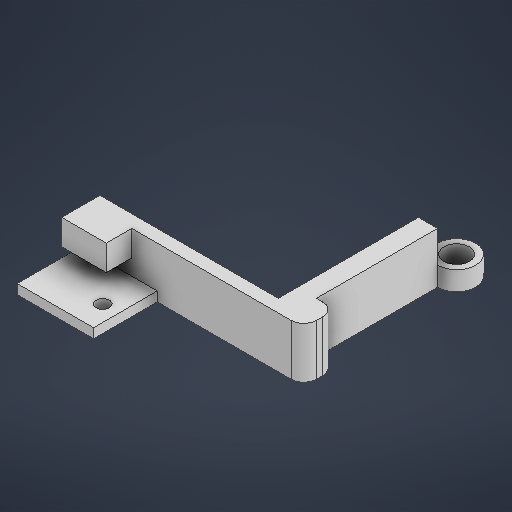
# Autodesk Inventor part: lewascianakoło
Saved by Autodesk Inventor 2026.2 (Build 302298010, 298A)
## iProperties
Created: 2026-04-27
Part Number: lewascianakoło
Material: Ogólny
Document SubType Name: Modeling
Designer: karol
Density: 1 g/cm^3
Appearance: Domyślna
Author: karol
Autodesk Inventor part; units mm, degrees
ref_plane "YZ Plane" through (0, 0, 0) normal (1, 0, 0) x (0, 1, 0)
ref_plane "XZ Plane" through (0, 0, 0) normal (0, 1, 0) x (-1, 0, 0)
ref_plane "XY Plane" through (0, 0, 0) normal (0, 0, 1) x (1, 0, 0)
sketch "Szkic1" plane through (0, 0, 0) normal (0, 1, 0) x (-1, 0, 0)
  line L0 (0, 0) -> (3, 0)
  line L1 (3, 0) -> (3, -25)
  line L2 (3, -25) -> (0, -25)
  line L3 (0, -25) -> (0, 0)
  line L4 (3, 0) -> (31, 0)
  line L5 (31, 0) -> (31, -3)
  line L6 (31, -3) -> (3, -3)
  line L7 (3, -3) -> (3, 0)
  point P0 (3, -3)
  dimension "d0" = 3
  dimension "d1" = 25
  dimension "d2" = 28
  dimension "d3" = 3
  constraints: 16 end point, 4 parallel, 2 horizontal, 2 perpendicular
  measures "d0" distance of L1.end L2.end
  measures "d1" distance of L0.end L1.end
  measures "d2" distance of L5.end L6.end
  measures "d3" distance of L4.end L5.end
extrude "Wyciągnięcie proste1" add sketch "Szkic1" along normal blind 8
sketch "Szkic7" plane through (0, 8, 0) normal (0, 1, 0) x (1, 0, 0)
  line L0 (-31, 0) -> (0, 0) projected
  line L1 (0, 0) -> (-3, 0)
  line L2 (-3, 0) -> (-3, 3)
  line L3 (-3, 3) -> (0, 3)
  line L4 (0, 3) -> (0, 0)
  line L5 (-3, 0) -> (3, 0)
  line L6 (3, 0) -> (3, 6)
  line L7 (3, 6) -> (-3, 6)
  line L8 (-3, 6) -> (-3, 0)
  circle A0 centre (0, 3) radius 1.5
  point P0 (-1.5, 3)
  point P1 (0, 1.5)
  dimension "d21" = 6
  dimension "d22" = 6
  dimension "d23" = 3
  constraints: 16 end point, 4 parallel, 2 horizontal, 2 perpendicular, 1 centre point, 1 coincident
  measures "d21" distance of L7.end L6.end
  measures "d22" distance of L6.end L5.end
  measures "d23" diameter of A0
extrude "Wyciągnięcie proste7" add sketch "Szkic7" against normal blind 8 contours L4 A0 L3 L8 L7 L6 L5
extrude "Wyciągnięcie proste8" cut sketch "Szkic7" against normal blind 8 contours A0 L3 L4 | L4 L3 A0
sketch "Szkic8" plane through (0, 8, 0) normal (0, 1, 0) x (1, 0, 0)
  circle A0 centre (0, 3) radius 1.5 projected
  circle A1 centre (0, 3) radius 2
  point P0 (0, 0)
  constraints: 1 centre point, 1 coincident
extrude "Wyciągnięcie proste9" add sketch "Szkic8" against normal blind 3 contours A0
sketch "Szkic9" plane through (0, 8, 0) normal (0, 1, 0) x (1, 0, 0)
  line L0 (-31, 3) -> (-31, 0) projected
  line L1 (3, 0) -> (3, 6) projected
  line L2 (-31, 0) -> (3, 0)
  line L3 (3, 0) -> (3, 1)
  line L4 (3, 1) -> (-31, 1)
  line L5 (-31, 1) -> (-31, 0)
  point P0 (0, 0)
  dimension "d30" = 1
  constraints: 8 end point, 2 parallel, 1 horizontal, 1 perpendicular, 1 point on line
  measures "d30" distance of L3.end L2.end
extrude "Wyciągnięcie proste10" cut sketch "Szkic9" against normal blind 8
sketch "Szkic10" plane through (0, 8, 0) normal (0, 1, 0) x (1, 0, 0)
  line L0 (0, 25) -> (-3, 25) projected
  line L1 (-3, 25) -> (3, 25)
  line L2 (3, 25) -> (3, 31)
  line L3 (3, 31) -> (-3, 31)
  line L4 (-3, 31) -> (-3, 25)
  point P0 (0, 0)
  dimension "d33" = 6
  dimension "d34" = 6
  constraints: 8 end point, 2 parallel, 1 horizontal, 1 perpendicular
  measures "d33" distance of L3.end L2.end
  measures "d34" distance of L2.end L1.end
extrude "Wyciągnięcie proste11" add sketch "Szkic10" against normal blind 8
sketch "Szkic11" plane through (0, 8, 0) normal (0, 1, 0) x (1, 0, 0)
  line L0 (3, 31) -> (3, 25) projected
  line L1 (3, 31) -> (-3, 31)
  line L2 (-3, 31) -> (-3, 25)
  line L3 (-3, 25) -> (3, 25)
  line L4 (3, 25) -> (3, 31)
  point P0 (0, 0)
  dimension "d37" = 6
  dimension "d38" = 6
  constraints: 8 end point, 2 parallel, 1 horizontal, 1 perpendicular
  measures "d37" distance of L3.end L2.end
  measures "d38" distance of L2.end L1.end
extrude "Wyciągnięcie proste12" cut sketch "Szkic11" against normal blind 5
sketch "Szkic12" plane through (0, 3, 0) normal (0, 1, 0) x (1, 0, 0)
  circle A0 centre (0, 28) radius 2
  line L0 (-3, 25) -> (-3, 31) projected
  line L1 (-3, 31) -> (3, 31) projected
  point P0 (0, 0)
  point P1 (-3, 28)
  point P2 (0, 31)
  dimension "d41" = 4
  dimension "d42" = 3
  dimension "d43" = 3
  constraints: 2 midpoint, 1 centre point
  measures "d41" diameter of A0
  measures "d42" distance of point (-3, 28) A0.centre
  measures "d43" distance of A0.centre point (0, 31)
extrude "Wyciągnięcie proste13" cut sketch "Szkic12" against normal blind 3
sketch "Szkic13" plane through (-31, 8, -1) normal (0, 0, 1) x (1, 0, 0)
  line L0 (0, 0) -> (7, 0)
  line L1 (7, 0) -> (7, -4)
  line L2 (7, -4) -> (0, -4)
  line L3 (0, -4) -> (0, 0)
  point P0 (31, -8)
  dimension "d46" = 7
  dimension "d47" = 4
  constraints: 8 end point, 2 parallel, 1 horizontal, 1 perpendicular
  measures "d46" distance of L1.end L2.end
  measures "d47" distance of L0.end L1.end
extrude "Wyciągnięcie proste14" add sketch "Szkic13" along normal blind 4
sketch "Szkic14" plane through (-31, 0, -3) normal (-1, 0, 0) x (0, 0, 1)
  circle A0 centre (4, 6) radius 1.5
  line L0 (2, 4) -> (6, 4) projected
  line L1 (6, 8) -> (6, 4) projected
  point P0 (3, 0)
  dimension "d50" = 3
  dimension "d51" = 2
  dimension "d52" = 2
  constraints: 1 centre point
  measures "d50" diameter of A0
  measures "d51" distance from line of L0 A0.centre
  measures "d52" distance from line of A0.centre L1
extrude "Wyciągnięcie proste15" cut sketch "Szkic14" against normal blind 6
sketch "Szkic15" plane through (-31, 0, -1) normal (0, 0, 1) x (1, 0, 0)
  line L0 (-1, 0) -> (11, 0)
  line L1 (11, 0) -> (11, 1.5)
  line L2 (11, 1.5) -> (-1, 1.5)
  line L3 (-1, 1.5) -> (-1, 0)
  point P0 (31, 0)
  dimension "d55" = 12
  dimension "d56" = 1.5
  constraints: 8 end point, 2 parallel, 1 horizontal, 1 perpendicular
  measures "d55" distance of L2.end L1.end
  measures "d56" distance of L1.end L0.end
extrude "Wyciągnięcie proste16" add sketch "Szkic15" along normal blind 10
sketch "Szkic16" plane through (-31, 1.5, -1) normal (0, 1, 0) x (1, 0, 0)
  circle A0 centre (8.5, -6.06) radius 1.05
  line L0 (7, 0) -> (34, 0) projected
  line L1 (-1, 0) -> (-1, -10) projected
  point P0 (31, -1)
  point P1 (0, 0)
  point P2 (-1, -10)
  dimension "d59" = 2.1
  dimension "d60" = 6.06
  dimension "d61" = 9.5
  constraints: 1 centre point, 1 other
  measures "d59" diameter of A0
  measures "d60" distance from line of L0 A0.centre
extrude "Wyciągnięcie proste17" cut sketch "Szkic16" against normal blind 2
fillet "Fillet1" radius 3 2 edges at (3, 1.5, -25) (3, 1.5, -31)
fillet "Fillet2" radius 2 2 edges at (3, 4, -1) (3, 4, -6)
fillet "Zaokrąglenie3" radius 3 1 edges at (-3, 1.5, -31)
